LinksPassive_v5 (Autodesk Fusion 360 design; units mm, degrees)
Autodesk Fusion 360 part; units mm, degrees
sketch "most" plane through (0, 0, 0) normal (0, 0, 1) x (1, 0, 0)
  line L0 (-18.5, 6) -> (-18.5, -6) construction
  line L1 (18.5, -6) -> (18.5, 6) construction
  line L2 (18.5, 6) -> (-18.5, -6) construction
  line L3 (-18.5, 6) -> (18.5, -6) construction
  circle A0 centre (12.5, 0) radius 0.95
  circle A1 centre (12.5, 0) radius 2.95
  circle A2 centre (12.5, 0) radius 6
  line L4 (0, 6) -> (0, -15) construction
  line L5 (12.5, 6) -> (0, 6)
  line L6 (0, -6) -> (12.5, -6)
  line L7 (12.5, -6) -> (12.5, 6)
  line L8 (12.5, 6) -> (-12.5, -6) construction
  line L9 (-12.5, 6) -> (12.5, -6) construction
  line L10 (18.5, 6) -> (0, 6) construction
  line L11 (-12.5, 6) -> (-18.5, 6) construction
  line L12 (-18.5, -6) -> (-12.5, -6) construction
  line L13 (0, -6) -> (18.5, -6) construction
  line L14 (0, -6) -> (-18.5, -6) construction
  line L15 (-12.5, -6) -> (-12.5, 6)
  line L16 (-18.5, 6) -> (0, 6) construction
  circle A3 centre (-12.5, 0) radius 6
  circle A4 centre (-12.5, 0) radius 2.95
  circle A5 centre (-12.5, 0) radius 0.95
  line L17 (0, -6) -> (-12.5, -6)
  line L18 (-12.5, 6) -> (0, 6)
  dimension "d2" = 12
  dimension "d3" = 1.9
  dimension "d4" = 5.9
  dimension "d5" = 12
  dimension "d6" = 12.5
  dimension "d7" = 25
  constraint horizontal L10
  constraint perpendicular L0 L10
  constraint parallel L10 L12
  constraint parallel L0 L1
  constraint coincident L2 origin
  constraint coincident L3 origin
  constraint concentric A0 A1
  constraint concentric A0 A2
  constraint perpendicular L4 L12
  constraint horizontal origin A0.centre
  constraint horizontal L5
  constraint parallel L5 L6
  constraint coincident A2 L5.start
  constraint coincident L8 origin
  constraint coincident L9 origin
  constraint collinear L10 L11
  constraint coincident L4 L6.start
  constraint collinear L12 L13
  constraint symmetric L1.end L4 L0.start
  constraint symmetric L1.start L4 L0.end
  constraint symmetric A0 L4 A5
  constraint symmetric A1 L4 A4
  constraint symmetric A2 L4 A3
  constraint symmetric L4 L5.start L9.start
  constraint symmetric L4 L6.end L8.end
  constraint symmetric L4 L5.end L10.end
  constraint symmetric L4 L6.start L13.start
  constraint perpendicular L15 L18
  measures "d2" distance of L0.start L0.end
  measures "d3" diameter of A0
  measures "d4" diameter of A1
  measures "d5" diameter of A2
  measures "d6" distance of origin A0.centre
  measures "d7" distance of L8.end L6.end
extrude "Extrude1" add sketch "most" along normal blind 10 contours A0 L7 | A0 A1 L7 | A1 A2 L7 | A2 L5 L6 A3 L17 L18 | L15 A3 A4 | L15 A4 A5 | L15 A5 picked at (12.1842, -0.0237) picked at (11.9703, -2.2146) picked at (10.0789, 4.3404) picked at (-7.547, -0.4246) picked at (-11.1532, -1.8368) picked at (-12.1866, 0.0451)
extrude "Extrude2" add sketch "most" along normal blind 12 contours A0 A1 L7 | A0 A1 L7 | A1 A2 L7 | A1 A2 L7
extrude "Extrude3" add sketch "most" along normal blind 17 contours A0 A1 L7 | A0 A1 L7
extrude "Extrude5" add sketch "most" against normal blind 2 contours L15 A3 A4 | L15 A3 A4 | L15 A4 A5 | L15 A4 A5
extrude "Extrude6" add sketch "most" against normal blind 7 contours L15 A4 A5 | L15 A4 A5
extrude "Extrude7" add sketch "most" along normal blind 10 contours L15 A3 A4 | L15 A4 A5 picked at (-14.9211, 4.3404) picked at (-13.0297, -2.2146)
extrude "Extrude8" cut sketch "most" along normal blind 10 and the other way blind 10 contours L15 A5 | L15 A5
extrude "Extrude9" cut sketch "most" along normal blind 17 contours A0 L7 | A0 L7
fillet "Fillet1" radius 0.3 1 edges at (9.7496, -1.0668, 17)
fillet "Fillet2" radius 0.3 1 edges at (-13.3857, -0.3435, -7)
sketch "top nut" plane through (0, 0, 10) normal (0, 0, 1) x (-1, 0, 0)
  arc A0 (12.5, -6) -> (12.5, 6) centre (12.5, 0) ccw
  line L0 (12.5, 6) -> (-12.5, 6)
  arc A1 (-12.5, -6) -> (-12.5, 6) centre (-12.5, 0) ccw
  line L1 (-12.5, -6) -> (12.5, -6)
  circle A2 centre (12.5, 0) radius 0.95
  circle A3 centre (12.5, 0) radius 2.5 construction
  line L2 (14.5842, -1.3806) -> (14.7377, 1.1147)
  line L3 (14.7377, 1.1147) -> (12.6535, 2.4953)
  line L4 (12.6535, 2.4953) -> (10.4158, 1.3806)
  line L5 (10.4158, 1.3806) -> (10.2623, -1.1147)
  line L6 (10.2623, -1.1147) -> (12.3465, -2.4953)
  line L7 (12.3465, -2.4953) -> (14.5842, -1.3806)
  point P0 (12.5, 0)
  dimension "d35" = 5
  constraint concentric A0 A3
  constraint coincident P0 A0.centre
  constraint coincident A3 L2.start
  measures "d35" diameter of A3
extrude "Extrude10" cut sketch "top nut" against normal blind 4 contours L2 L3 L4 L5 L6 L7
sketch "bottom nut" plane through (0, 0, 0) normal (0, 0, -1) x (1, 0, 0)
  circle A0 centre (12.5, 0) radius 0.95
  arc A1 (-12.5, -6) -> (-12.5, 6) centre (-12.5, 0) ccw
  line L0 (-12.5, -6) -> (12.5, -6)
  arc A2 (12.5, -6) -> (12.5, 6) centre (12.5, 0) ccw
  line L1 (12.5, 6) -> (-12.5, 6)
  circle A3 centre (12.5, 0) radius 2.5 construction
  line L2 (10, 1.4434) -> (10, -1.4434)
  line L3 (10, -1.4434) -> (12.5, -2.8868)
  line L4 (12.5, -2.8868) -> (15, -1.4434)
  line L5 (15, -1.4434) -> (15, 1.4434)
  line L6 (15, 1.4434) -> (12.5, 2.8868)
  line L7 (12.5, 2.8868) -> (10, 1.4434)
  point P0 (12.5, 0)
  dimension "d38" = 5
  constraint concentric A0 A3
  constraint coincident P0 A0.centre
  constraint vertical L3.end P0
  measures "d38" diameter of A3
extrude "Extrude11" cut sketch "bottom nut" against normal blind 4 contours L2 L3 L4 L5 L6 L7
fillet "Fillet3" radius 0.3 1 edges at (-15.2504, 1.0668, -7)
move_body "Move2" bodies 1 to x (1, 0, 0) y (0, 1, 0) z (0, 0, 1) at (0, 0, 7)
equation "d25 = 0.0 °"
